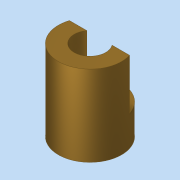
# Autodesk Inventor part: ShaftCollar
Saved by Autodesk Inventor 2017 (Build 210142000, 142)
## iProperties
Created: 2017-11-01
Part Number: ShaftCollar
Material: Brass, Soft Yellow
Document SubType Name: Modeling
Designer: Derek Wider
Density: 8.47 g/cm^3
Appearance: Brass - Satin
Author: Derek Wider
Autodesk Inventor part; units mm, degrees
ref_plane "YZ Plane" through (0, 0, 0) normal (1, 0, 0) x (0, 1, 0)
ref_plane "XZ Plane" through (0, 0, 0) normal (0, 1, 0) x (-1, 0, 0)
ref_plane "XY Plane" through (0, 0, 0) normal (0, 0, 1) x (1, 0, 0)
sketch "Sketch1" plane through (0, 0, 0) normal (0, 1, 0) x (-1, 0, 0)
  circle A0 centre (0, 0) radius 1.5875
  circle A1 centre (0, 0) radius 3.175
  dimension "d0" = 3.175
  dimension "d1" = 6.35
  constraints: 2 centre point, 2 coincident
  measures "d0" diameter of A0
  measures "d1" diameter of A1
extrude "Extrusion1" add sketch "Sketch1" along normal blind 8.128
sketch "Sketch2" plane through (0, 8.128, 0) normal (0, 1, 0) x (1, 0, 0)
  line L0 (-3.175, 3.7564) -> (3.175, 3.7564)
  line L1 (3.175, 3.7564) -> (3.175, 0.9525)
  line L2 (3.175, 0.9525) -> (-3.175, 0.9525)
  line L3 (-3.175, 0.9525) -> (-3.175, 3.7564)
  point P0 (0, 0)
  dimension "d4" = 3.175
  dimension "d5" = 6.35
  dimension "d6" = 0.9525
  constraints: 8 end point, 2 parallel, 1 horizontal, 1 perpendicular
  measures "d4" horizontal distance of point (0, 0) L1.end
  measures "d5" distance of L0.start L0.end
  measures "d6" distance from line of point (0, 0) L2
extrude "Extrusion2" cut sketch "Sketch2" against normal blind 5.08
body "Solid1"
